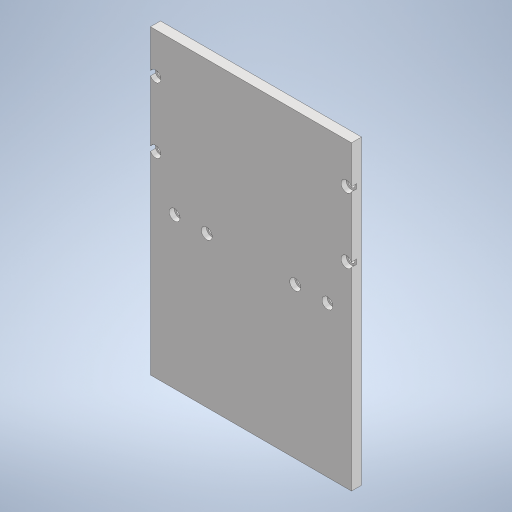
# Autodesk Inventor part: 200x300(10li)
Saved by Autodesk Inventor 2023 (Build 270158000, 158)
## iProperties
Created: 2025-04-11
Part Number: 200x300(10li)
Material: Generic
Document SubType Name: Modeling
Designer: huyqu
Density: 1 g/cm^3
Appearance: Default
Author: huyqu
Autodesk Inventor part; units mm, degrees
ref_plane "YZ Plane" through (0, 0, 0) normal (1, 0, 0) x (0, 1, 0)
ref_plane "XZ Plane" through (0, 0, 0) normal (0, 1, 0) x (-1, 0, 0)
ref_plane "XY Plane" through (0, 0, 0) normal (0, 0, 1) x (1, 0, 0)
sketch "Sketch1" plane through (0, 0, 0) normal (0, 0, 1) x (1, 0, 0)
  line L0 (0, 0) -> (200, 0)
  line L1 (200, 0) -> (200, 300)
  line L2 (200, 300) -> (0, 300)
  line L3 (0, 300) -> (0, 0)
  dimension "d0" = 200
  dimension "d1" = 300
  constraints: 8 end point, 2 parallel, 1 horizontal, 1 perpendicular
  measures "d0" distance of L0.start L0.end
  measures "d1" distance of L0.end L1.end
extrude "Extrusion1" add sketch "Sketch1" along normal blind 10
sketch "Sketch2" plane through (0, 0, 10) normal (0, 0, 1) x (1, 0, 0)
  circle A0 centre (5, 195) radius 2.4585 projected
  line L0 (0, 300) -> (0, 0) projected
  circle A1 centre (5, 260) radius 2.4585 projected
  circle A2 centre (195, 260) radius 2.4585 projected
  circle A3 centre (195, 195) radius 2.4585 projected
hole "Hole1" at (195, 195, 10) at (195, 260, 10) at (5, 195, 10) at (5, 260, 10) direction (0, 0, -1) diameter 7 end through all counterbore diameter 11 counterbore depth 5
sketch "Sketch3" plane through (0, 0, 10) normal (0, 0, 1) x (1, 0, 0)
  circle A0 centre (24, 150) radius 2.4585 projected
  circle A1 centre (24, 150) radius 2.4585 projected
  circle A2 centre (56, 150) radius 2.4585 projected
  circle A3 centre (144, 150) radius 2.4585 projected
  circle A4 centre (176, 150) radius 2.4585 projected
  point P0 (0, 0)
hole "Hole2" at (176, 150, 10) at (144, 150, 10) at (56, 150, 10) at (24, 150, 10) direction (0, 0, -1) diameter 7 end through all counterbore diameter 11 counterbore depth 5
body "Solid1"
